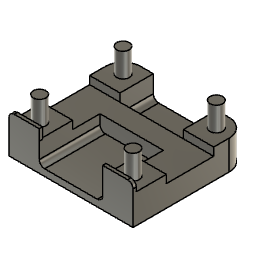
Smolboat Cutiepie (Seilboat) USB Port Insert (Autodesk Fusion 360 design; units mm, degrees)
Autodesk Fusion 360 part; units mm, degrees
sketch "USB Port Insert" plane through (0, 0, 0) normal (0, 0, 1) x (1, 0, 0)
  line L0 (90.2, -56.176) -> (90.2, -61.176)
  line L1 (90.2, -61.176) -> (85.65, -61.176)
  line L2 (85.65, -56.176) -> (90.2, -56.176)
  line L3 (85.65, -61.176) -> (85.65, -56.176)
  line L4 (90.2, -56.176) -> (90.2, -44.076)
  line L5 (99.7, -44.076) -> (99.7, -56.176)
  line L6 (99.7, -56.176) -> (90.2, -56.176)
  line L7 (90.2, -44.076) -> (99.7, -44.076)
  line L8 (85.65, -49.076) -> (90.2, -49.076)
  line L9 (90.2, -49.076) -> (90.2, -56.176)
  line L10 (90.2, -56.176) -> (85.65, -56.176)
  line L11 (85.65, -56.176) -> (85.65, -49.076)
  line L12 (104.25, -49.076) -> (104.25, -56.176)
  line L13 (99.7, -56.176) -> (99.7, -49.076)
  line L14 (104.25, -56.176) -> (99.7, -56.176)
  line L15 (99.7, -49.076) -> (104.25, -49.076)
  circle A0 centre (87.95, -46.376) radius 0.95
  circle A1 centre (87.95, -58.876) radius 0.95
  circle A2 centre (101.95, -46.376) radius 0.95
  circle A3 centre (101.95, -58.876) radius 0.95
  line L16 (90.2, -49.076) -> (85.65, -49.076)
  line L17 (85.65, -49.076) -> (85.65, -46.776)
  spline S0 degree 3 poles (85.65, -46.776) (85.65, -45.2848) (86.8588, -44.076) (88.35, -44.076) knots 2 2 2 2 3 3 3 3
  line L18 (88.35, -44.076) -> (90.2, -44.076)
  line L19 (90.2, -44.076) -> (90.2, -49.076)
  line L20 (99.7, -49.076) -> (104.25, -49.076)
  line L21 (104.25, -49.076) -> (104.25, -46.776)
  spline S1 degree 3 poles (104.25, -46.776) (104.25, -45.2848) (103.0412, -44.076) (101.55, -44.076) knots 2 2 2 2 3 3 3 3
  line L22 (101.55, -44.076) -> (99.7, -44.076)
  line L23 (99.7, -44.076) -> (99.7, -49.076)
  line L24 (99.7, -56.176) -> (104.25, -56.176)
  line L25 (104.25, -56.176) -> (104.25, -61.176)
  line L26 (104.25, -61.176) -> (99.7, -61.176)
  line L27 (99.7, -61.176) -> (99.7, -56.176)
  line L28 (99.7, -61.176) -> (90.2, -61.176)
  line L29 (99.7, -56.176) -> (99.7, -61.176)
  line L30 (90.2, -61.176) -> (90.2, -56.176)
  line L31 (90.2, -56.176) -> (99.7, -56.176)
extrude "Extrude1" add sketch "USB Port Insert" along normal blind 1 contours L0 L6 L27 L28 L29 L30 L31
extrude "Extrude2" add sketch "USB Port Insert" along normal blind 1 contours L4 L5 L6 L7 L9 L13 L19 L23 L31
extrude "Extrude3" add sketch "USB Port Insert" along normal blind 3.2 contours L2 L4 L8 L9 L10 L11 L16
extrude "Extrude4" add sketch "USB Port Insert" along normal blind 3.2 contours L5 L12 L13 L14 L15 L20 L24
extrude "Extrude5" add sketch "USB Port Insert" along normal blind 4.2 contours L5 L15 L20 L21 S1 L22 L23
extrude "Extrude6" add sketch "USB Port Insert" along normal blind 4.2 contours L4 L8 L16 L17 S0 L18 L19
extrude "Extrude7" add sketch "USB Port Insert" along normal blind 4.2 contours L0 L1 L2 L3 L10 L30
extrude "Extrude8" add sketch "USB Port Insert" along normal blind 4.2 contours L14 L24 L25 L26 L27 L29
extrude "Extrude9" add sketch "USB Port Insert" along normal blind 8 contours A0
extrude "Extrude10" add sketch "USB Port Insert" along normal blind 8 contours A2
extrude "Extrude11" add sketch "USB Port Insert" along normal blind 8 contours A1
extrude "Extrude12" add sketch "USB Port Insert" along normal blind 8 contours A3
ref_plane "WorkPlane1" through (94.95, -61.176, 2.1) normal (0, -1, 0) x (1, 0, 0)
sketch "Layer 2" plane through (0, -61.176, 0) normal (0, -1, 0) x (-1, 0, 0)
  line L0 (-99.7, -5.8) -> (-99.7, -1.8)
  spline S0 degree 3 poles (-99.7, -1.8) (-99.7, -1.3582) (-99.3418, -1) (-98.9, -1) knots 1 1 1 1 2 2 2 2
  line L1 (-98.9, -1) -> (-91, -1)
  spline S1 degree 3 poles (-91, -1) (-90.5582, -1) (-90.2, -1.3582) (-90.2, -1.8) knots 3 3 3 3 4 4 4 4
  line L2 (-90.2, -1.8) -> (-90.2, -5.8)
  line L3 (-90.2, -5.8) -> (-86.45, -5.8)
  spline S2 degree 3 poles (-86.45, -5.8) (-86.0082, -5.8) (-85.65, -5.4418) (-85.65, -5) knots 6 6 6 6 7 7 7 7
  line L4 (-85.65, -5) -> (-85.65, 0)
  line L5 (-85.65, 0) -> (-104.25, 0)
  line L6 (-104.25, 0) -> (-104.25, -5)
  spline S3 degree 3 poles (-104.25, -5) (-104.25, -5.4418) (-103.8918, -5.8) (-103.45, -5.8) knots 10 10 10 10 11 11 11 11
  line L7 (-103.45, -5.8) -> (-99.7, -5.8)
extrude "Extrude13" add sketch "Layer 2" against normal blind 1
extrude "Extrude14" cut 1 faces at (87.4333, -60.176, 4.7333) along direction (0, -1, 0) blind 0.5
extrude "Extrude15" cut 1 faces at (102.4667, -60.176, 4.7333) along direction (0, -1, 0) blind 0.5
extrude "Extrude16" add 1 faces at (99.5382, -60.176, 1.1526) along direction (0, 1, 0) blind 16.5
extrude "Extrude17" add 1 faces at (90.3526, -60.176, 1.1618) along direction (0, 1, 0) blind 16.5
extrude "Extrude18" cut 1 faces at (90.2, -43.9427, 1.5333) along direction (1, 0, 0) blind 1.6
extrude "Extrude19" cut 1 faces at (99.7, -43.9427, 1.2667) along direction (-1, 0, 0) blind 1.1
extrude "Extrude20" add 1 faces at (101.9903, -56.7602, 4.2) along direction (0, 0, 1) blind 0.2
extrude "Extrude21" add 1 faces at (87.9097, -56.7602, 4.2) along direction (0, 0, 1) blind 0.2
extrude "Extrude22" add 1 faces at (87.9097, -48.4918, 4.2) along direction (0, 0, 1) blind 0.2
extrude "Extrude23" add 1 faces at (101.9903, -48.4918, 4.2) along direction (0, 0, 1) blind 0.2
sketch "block" plane through (104.25, 0, 0) normal (1, 0, 0) x (0, 1, 0)
  line L0 (-49.076, 0) -> (-52.076, 0)
  line L1 (-49.076, 3.2) -> (-49.076, 0)
  line L2 (-52.076, 3.2) -> (-49.076, 3.2)
  line L3 (-52.076, 0) -> (-52.076, 3.2)
extrude "Extrude24" add sketch "block" against normal blind 17.5
